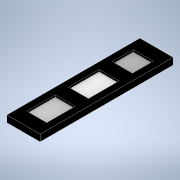
# Autodesk Inventor part: LED
Saved by Autodesk Inventor 2021 (Build 250183000, 183)
## iProperties
Created: 2024-06-13
Part Number: LED
Material: PC/ABS Plastic
Document SubType Name: Modeling
Designer: ASUS
Density: 0.357273 g/cm^3
Appearance: Anodized - Black
Author: ASUS
Autodesk Inventor part; units mm, degrees
ref_plane "YZ Plane" through (0, 0, 0) normal (1, 0, 0) x (0, 1, 0)
ref_plane "XZ Plane" through (0, 0, 0) normal (0, 1, 0) x (-1, 0, 0)
ref_plane "XY Plane" through (0, 0, 0) normal (0, 0, 1) x (1, 0, 0)
sketch "Sketch1" plane through (0, 0, 0) normal (0, 1, 0) x (-1, 0, 0)
  line L0 (0, 0) -> (50, 0)
  line L1 (50, 0) -> (50, -200)
  line L2 (50, -200) -> (0, -200)
  line L3 (0, -200) -> (0, 0)
  dimension "d0" = 50
  dimension "d1" = 200
  constraints: 8 end point, 2 parallel, 1 horizontal, 1 perpendicular
  measures "d0" distance between parallel lines of L3 L1
  measures "d1" distance between parallel lines of L2 L0
extrude "Extrusion1" add sketch "Sketch1" along normal blind 10
sketch "Sketch2" plane through (0, 10, 0) normal (0, 1, 0) x (1, 0, 0)
  line L0 (-40, 180) -> (-10, 180)
  line L1 (-10, 180) -> (-10, 148.7634)
  line L2 (-10, 148.7634) -> (-40, 148.7634)
  line L3 (-40, 148.7634) -> (-40, 180)
  line L4 (-40, 128.7634) -> (-10, 128.7634)
  line L5 (-10, 128.7634) -> (-10, 82.7005)
  line L6 (-10, 82.7005) -> (-40, 82.7005)
  line L7 (-40, 82.7005) -> (-40, 128.7634)
  line L8 (-40, 62.7005) -> (-10, 62.7005)
  line L9 (-10, 62.7005) -> (-10, 20)
  line L10 (-10, 20) -> (-40, 20)
  line L11 (-40, 20) -> (-40, 62.7005)
  line L12 (0, 200) -> (-50, 200) projected
  line L13 (-50, 0) -> (0, 0) projected
  line L14 (-50, 200) -> (-50, 0) projected
  line L15 (0, 0) -> (0, 200) projected
  dimension "d4" = 20
  dimension "d5" = 20
  dimension "d6" = 20
  dimension "d7" = 20
  dimension "d8" = 10
  dimension "d9" = 10
  dimension "d10" = 10
  dimension "d11" = 10
  constraints: 24 end point, 6 parallel, 3 horizontal, 3 perpendicular, 3 point on line
  measures "d4" distance between parallel lines of L0 L12
  measures "d5" distance between parallel lines of L4 L2
  measures "d6" distance between parallel lines of L6 L8
  measures "d7" distance between parallel lines of L13 L10
  measures "d8" distance between parallel lines of L14 L3
  measures "d9" distance between parallel lines of L14 L7
  measures "d10" distance between parallel lines of L15 L1
  measures "d11" distance between parallel lines of L15 L5
extrude "Extrusion2" cut sketch "Sketch2" against normal blind 3 contours L0 L1 L2 L3 | L4 L5 L6 L7 | L8 L9 L10 L11
body "Solid1"
